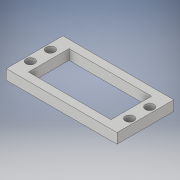
# Autodesk Inventor part: МД.001.1002 - Направляющие
Saved by Autodesk Inventor 2019 (Build 230136000, 136)
## iProperties
Created: 2019-12-30
Part Number: МД.001.1002 - Направляющие
Material: Типовые
Document SubType Name: Modeling
Designer: Петров Иван
Density: 1 g/cm^3
Appearance: По умолчанию
Author: Петров Иван
Autodesk Inventor part; units mm, degrees
ref_plane "YZ Plane" through (0, 0, 0) normal (1, 0, 0) x (0, 1, 0)
ref_plane "XZ Plane" through (0, 0, 0) normal (0, 1, 0) x (-1, 0, 0)
ref_plane "XY Plane" through (0, 0, 0) normal (0, 0, 1) x (1, 0, 0)
sketch "Эскиз1" plane through (0, 0, 0) normal (0, 1, 0) x (-1, 0, 0)
  line L0 (-10, -10) -> (-10, 10)
  line L1 (-10, 10) -> (-16, 10)
  arc A0 (-16, 10) -> (-17, 9) centre (-16, 9) ccw
  line L2 (-17, 9) -> (-17, 6.15)
  line L3 (-17, 6.15) -> (-15.934, 6.15)
  arc A1 (-15.934, 3.75) -> (-15.934, 6.15) centre (-14.15, 4.95) ccw
  line L4 (-15.934, 3.75) -> (-17, 3.75)
  line L5 (-17, 3.75) -> (-17, -3.75)
  line L6 (-17, -3.75) -> (-15.934, -3.75)
  arc A2 (-15.934, -6.15) -> (-15.934, -3.75) centre (-14.15, -4.95) ccw
  line L7 (-15.934, -6.15) -> (-17, -6.15)
  line L8 (-17, -6.15) -> (-17, -9)
  arc A3 (-17, -9) -> (-16, -10) centre (-16, -9) ccw
  line L9 (-16, -10) -> (-10, -10)
  line L10 (37.7, -3.75) -> (36.634, -3.75)
  line L11 (37.7, 3.75) -> (37.7, -3.75)
  line L12 (36.634, 3.75) -> (37.7, 3.75)
  arc A4 (36.634, 6.15) -> (36.634, 3.75) centre (34.85, 4.95) ccw
  line L13 (37.7, 6.15) -> (36.634, 6.15)
  line L14 (37.7, 9) -> (37.7, 6.15)
  arc A5 (37.7, 9) -> (36.7, 10) centre (36.7, 9) ccw
  line L15 (30.7, 10) -> (36.7, 10)
  line L16 (30.7, -10) -> (30.7, 10)
  line L17 (36.7, -10) -> (30.7, -10)
  arc A6 (36.7, -10) -> (37.7, -9) centre (36.7, -9) ccw
  line L18 (37.7, -6.15) -> (37.7, -9)
  line L19 (36.634, -6.15) -> (37.7, -6.15)
  arc A7 (36.634, -3.75) -> (36.634, -6.15) centre (34.85, -4.95) ccw
  line L20 (-10, 10) -> (30.7, 10)
  line L21 (30.7, -10) -> (-10, -10)
  line L22 (-10, -10) -> (-10, 10)
  circle A8 centre (0, 0) radius 1.25
  circle A9 centre (0, 0) radius 3.4957
  circle A10 centre (0, 0) radius 2.6787
  circle A11 centre (0, 0) radius 5.4
  line L23 (37.7, 6.15) -> (37.7, 3.75)
  line L24 (37.7, -3.75) -> (37.7, -6.15)
  line L25 (37.7, 3.75) -> (37.7, 0.5)
  line L26 (-17, 3.75) -> (-17, -3.75)
  line L27 (-17, 6.15) -> (-17, 3.75)
  line L28 (-17, 3.75) -> (-17, -3.75)
  line L29 (-17, -3.75) -> (-17, -6.15)
  circle A12 centre (-14.15, 4.95) radius 2.15
  circle A13 centre (-14.15, -4.95) radius 2.15
  arc A14 (36.634, -3.75) -> (36.634, -6.15) centre (34.85, -4.95) ccw
  circle A15 centre (34.85, -4.95) radius 2.15
  circle A16 centre (34.85, 4.95) radius 2.15
  line L30 (37.7, 9) -> (37.7, 14)
  line L31 (37.7, 14) -> (-17, 14)
  line L32 (-17, 14) -> (-17, 9)
  line L33 (37.7, -9) -> (37.7, -14)
  line L34 (37.7, -14) -> (-17, -14)
  line L35 (-17, -14) -> (-17, -9)
  point P0 (10.35, -10)
  dimension "d0" = 5
  dimension "d1" = 5
  constraints: 72 end point, 18 point on circle, 16 centre point, 4 coincident, 4 collinear, 4 point on line, 2 concentric, 2 perpendicular, 2 vertical, 3 other
  measures "d0" distance of L14.start L30.end
  measures "d1" distance of L18.end L33.end
extrude "Выдавливание1" add sketch "Эскиз1" along normal blind 5 contours L9 A3 L8 L7 A2 L6 L5 L4 A1 L3 L2 A0 L1 L0 | L21 L17 A6 L33 L34 L35 A3 L9 | L1 A0 L32 L31 L30 A5 L15 L20 | L16 L15 A5 L14 L13 A4 L12 L11 L10 A7 L19 L18 A6 L17 | L29 L6 A13 L7 | L3 A12 L4 L27 | L19 A15 L10 L24 | L23 L12 A16 L13
